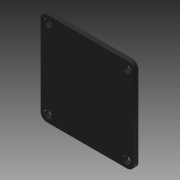
# Autodesk Inventor part: FC 36x36
Saved by Autodesk Inventor 2015 (Build 190159000, 159)
## iProperties
Created: 2016-11-27
Part Number: FC 36x36
Material: Generic
Document SubType Name: Modeling
Designer: Hampus
Density: 1 g/cm^3
Appearance: Rubber - Black
Author: Hampus
Autodesk Inventor part; units mm, degrees
note: some values were not read from the file. Chosen so that the rebuilt part matches the saved one: sketch regions of "Extrusion3".
ref_plane "YZ Plane" through (0, 0, 0) normal (1, 0, 0) x (0, 1, 0)
ref_plane "XZ Plane" through (0, 0, 0) normal (0, 1, 0) x (-1, 0, 0)
ref_plane "XY Plane" through (0, 0, 0) normal (0, 0, 1) x (1, 0, 0)
sketch "Sketch1" plane through (0, 0, 0) normal (0, 1, 0) x (-1, 0, 0)
  line L0 (-2.5, 0) -> (-33.5, 0)
  line L1 (-36, -2.5) -> (-36, -33.5)
  line L2 (-33.5, -36) -> (-2.5, -36)
  line L3 (0, -33.5) -> (0, -2.5)
  line L4 (-10.5351, -31.1412) -> (-23.3582, -31.1412)
  line L5 (-23.3582, -31.1412) -> (-23.3582, -27.4511)
  line L6 (-23.3582, -27.4511) -> (-10.5351, -27.4511)
  line L7 (-10.5351, -27.4511) -> (-10.5351, -31.1412)
  line L8 (-9.059, -24.6835) -> (-4.3542, -24.6835)
  line L9 (-4.3542, -24.6835) -> (-4.3542, -15.1815)
  line L10 (-4.3542, -15.1815) -> (-9.059, -15.1815)
  line L11 (-9.059, -15.1815) -> (-9.059, -24.6835)
  line L12 (-9.059, -9.1851) -> (-14.6864, -9.1851)
  line L13 (-14.6864, -9.1851) -> (-14.6864, -4.2957)
  line L14 (-14.6864, -4.2957) -> (-9.059, -4.2957)
  line L15 (-9.059, -4.2957) -> (-9.059, -9.1851)
  line L16 (-12.3801, -22.1005) -> (-25.2032, -22.1005)
  line L17 (-25.2032, -22.1005) -> (-25.2032, -13.3365)
  line L18 (-25.2032, -13.3365) -> (-12.3801, -13.3365)
  line L19 (-12.3801, -13.3365) -> (-12.3801, -22.1005)
  line L20 (-23.3582, -8.5394) -> (-29.1701, -8.5394)
  line L21 (-29.1701, -8.5394) -> (-29.1701, -3.4445)
  line L22 (-29.1701, -3.4445) -> (-23.3582, -3.4445)
  line L23 (-23.3582, -3.4445) -> (-23.3582, -8.5394)
  line L24 (-32.5555, -15.1815) -> (-29.1701, -15.1815)
  line L25 (-29.1701, -15.1815) -> (-29.1701, -21.2702)
  line L26 (-29.1701, -21.2702) -> (-32.5555, -21.2702)
  line L27 (-32.5555, -21.2702) -> (-32.5555, -15.1815)
  line L28 (-30.8628, -27.4511) -> (-29.1701, -27.4511)
  line L29 (-29.1701, -27.4511) -> (-29.1701, -25.9751)
  line L30 (-29.1701, -25.9751) -> (-30.8628, -25.9751)
  line L31 (-30.8628, -25.9751) -> (-30.8628, -27.4511)
  line L32 (-25.2032, -25.9751) -> (-23.3582, -25.9751)
  line L33 (-23.3582, -25.9751) -> (-23.3582, -24.6835)
  line L34 (-23.3582, -24.6835) -> (-25.2032, -24.6835)
  line L35 (-25.2032, -24.6835) -> (-25.2032, -25.9751)
  line L36 (-16.9466, -25.9751) -> (-15.609, -25.9751)
  line L37 (-15.609, -25.9751) -> (-15.609, -23.8533)
  line L38 (-15.609, -23.8533) -> (-16.9466, -23.8533)
  line L39 (-16.9466, -23.8533) -> (-16.9466, -25.9751)
  line L40 (-6.7066, -31.1412) -> (-5.2767, -31.1412)
  line L41 (-5.2767, -31.1412) -> (-5.2767, -29.2962)
  line L42 (-5.2767, -29.2962) -> (-6.7066, -29.2962)
  line L43 (-6.7066, -29.2962) -> (-6.7066, -31.1412)
  line L44 (-7.214, -11.6759) -> (-1.9445, -11.6759)
  line L45 (-1.9445, -11.6759) -> (-1.9445, -10.5689)
  line L46 (-1.9445, -10.5689) -> (-7.214, -10.5689)
  line L47 (-7.214, -10.5689) -> (-7.214, -11.6759)
  line L48 (0, -18) -> (-36, -18)
  line L49 (-18, -36) -> (-18, 0)
  circle A0 centre (-2.75, -33.25) radius 1.5
  circle A1 centre (-33.25, -33.25) radius 1.5
  circle A2 centre (-33.25, -2.75) radius 1.5
  circle A3 centre (-2.75, -2.75) radius 1.5
  arc A4 (-2.5, -36) -> (0, -33.5) centre (-2.5, -33.5) ccw
  arc A5 (-36, -33.5) -> (-33.5, -36) centre (-33.5, -33.5) ccw
  arc A6 (-33.5, 0) -> (-36, -2.5) centre (-33.5, -2.5) ccw
  arc A7 (0, -2.5) -> (-2.5, 0) centre (-2.5, -2.5) ccw
  point P0 (0, 0)
  point P1 (-36, -36)
  point P2 (-36, 0)
  point P3 (0, -36)
  dimension "d0" = 36
  dimension "d1" = 36
  dimension "d13" = 3
  dimension "d14" = 3
  dimension "d15" = 3
  dimension "d16" = 3
  dimension "d17" = 2.5
  constraints: 100 end point, 24 parallel, 20 point on line, 12 horizontal, 12 perpendicular, 8 centre point, 8 point on circle, 8 tangent, 4 midpoint, 3 equal radius
  measures "d0" distance of point (0, -36) point (-36, -36)
  measures "d1" distance of point (-36, -36) point (-36, 0)
  measures "d13" diameter of A0
  measures "d14" diameter of A1
  measures "d15" diameter of A2
  measures "d16" diameter of A3
  measures "d17" radius of A4
extrude "Extrusion2" add sketch "Sketch1" along normal blind 2.2 contours L49 L48 L17 L18 | L18 L19 L48 L49 | L49 L16 L17 L48 | L48 L19 L16 L49 | L48 L11 L10 L9 | L9 L8 L11 L48 | L48 L25 L26 L27 | L27 L24 L25 L48 | L49 L4 L5 L6 | L6 L7 L4 L49 | L12 L13 L14 L15 | L20 L21 L22 L23 | L31 L30 L29 L28 | L35 L34 L33 L32 | L39 L38 L37 L36 | L43 L42 L41 L40 | L47 L46 L45 L44
extrude "Extrusion3" add sketch "Sketch1" along normal blind 1.8 contours A7 L3 L48 L9 L10 L11 L19 L18 L49 L0 | L49 L18 L17 L48 L25 L24 L27 L1 A6 L0 | L49 L48 L17 L18 | L18 L19 L48 L49 | L3 A4 L2 L49 L4 L7 L6 L16 L19 L48 L11 L8 L9 | L49 L16 L17 L48 | L48 L19 L16 L49 | L48 L27 L26 L25 L17 L16 L49 L6 L5 L4 L2 A5 L1
body "Solid1"
